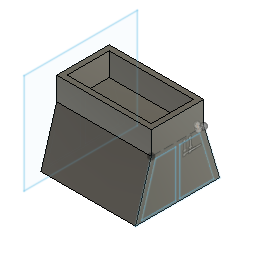
creality-ender-3-v2-foot-extender (Autodesk Fusion 360 design; units mm, degrees)
Autodesk Fusion 360 part; units mm, degrees
sketch "Sketch1" plane through (0, 0, 0) normal (0, 0, 1) x (1, 0, 0)
  line L0 (20, -10) -> (-20, -10)
  line L1 (-20, -10) -> (-20, 10)
  line L2 (-20, 10) -> (20, 10)
  line L3 (20, 10) -> (20, -10)
  line L4 (20, -10) -> (-20, 10) construction
  line L5 (-20, -10) -> (20, 10) construction
  line L6 (22.5, -12.5) -> (-22.5, -12.5)
  line L7 (-22.5, -12.5) -> (-22.5, 12.5)
  line L8 (-22.5, 12.5) -> (22.5, 12.5)
  line L9 (22.5, 12.5) -> (22.5, -12.5)
  line L10 (22.5, -12.5) -> (-22.5, 12.5) construction
  line L11 (-22.5, -12.5) -> (22.5, 12.5) construction
  dimension "d1" = 40
  dimension "d2" = 20
  dimension "d3" = 45
  dimension "d4" = 25
  constraint horizontal L0
  constraint perpendicular L0 L1
  constraint parallel L0 L2
  constraint parallel L1 L3
  constraint coincident L4 origin
  constraint coincident L5 origin
  constraint horizontal L6
  constraint perpendicular L6 L7
  constraint parallel L6 L8
  constraint parallel L7 L9
  constraint coincident L10 origin
  constraint coincident L11 origin
  measures "d1" distance of L1.end L2.end
  measures "d2" distance of L0.end L1.end
  measures "d3" distance of L7.end L8.end
  measures "d4" distance of L6.end L7.end
extrude "Extrude1" add sketch "Sketch1" along normal blind 11 makes body 1
sketch "Sketch4" plane through (22.5, 0, 0) normal (1, 0, 0) x (0, 1, 0)
  line L0 (-12.5, 0) -> (12.5, 0)
  line L1 (12.5, 0) -> (12.5, 11)
  line L2 (12.5, 11) -> (-12.5, 11)
  line L3 (-12.5, 11) -> (-12.5, 0)
  line L4 (-12.5, 0) -> (12.281, 0) construction
  line L5 (-12.5, 0) -> (-20, -25)
  line L6 (-20, -25) -> (20, -25)
  line L7 (20, -25) -> (12.5, 0)
  line L8 (12.5, 0) -> (20, -25) construction
  line L9 (12.281, -0.0657) -> (12.5, 0) construction
  line L10 (-12.5, 0) -> (-20, -25) construction
  line L11 (17.0904, -24.0014) -> (10.4521, -1.8738)
  line L12 (-17.0895, -23.9987) -> (-10.4636, -1.8738) construction
  line L13 (-1, -1.8738) -> (-1, -24)
  line L14 (1, -24.0002) -> (1, -1.8738)
  line L15 (-17.0895, -23.9987) -> (-1, -24)
  line L16 (1, -24.0002) -> (17.0904, -24.0014)
  line L17 (17.0904, -24.0014) -> (10.4521, -1.8738) construction
  line L18 (9.8899, 0) -> (9.2425, 2.1581) construction
  line L19 (-17.0895, -23.9987) -> (-10.4636, -1.8738)
  line L20 (-10.4636, -1.8738) -> (-1, -1.8738)
  line L21 (1, -1.8738) -> (10.4521, -1.8738)
  constraint horizontal L4
  constraint coincident L0.start L3.end
  constraint coincident L0.end L1.start
  constraint perpendicular L4 L14
  constraint collinear L15 L16
  constraint coincident L4 L18.start
  constraint collinear L17 L18
  constraint horizontal L20
  constraint coincident L14.end L20
  constraint collinear L20 L21
  constraint vertical L13
extrude "Extrude10" add sketch "Sketch4" against normal blind 2 separate body contours L11 L14 L16 L21 | L13 L15 L19 L20 makes body 2 at (22.5, 9.5141, -16.6251) makes body 3 at (22.5, -9.5177, -16.6242)
extrude "Extrude8" add sketch "Sketch4" against normal up to surface (45 mm away) contours L0 L5 L6 L7 bodies 1
sketch "Sketch9" plane through (0, 0, -1.8738) normal (0, 0, -1) x (1, 0, 0)
  line L0 (-22.5, 10.4636) -> (-22.5, 1)
  line L1 (-22.5, 1) -> (22.5, 1)
  line L2 (22.5, 1) -> (22.5, 10.4636)
  line L3 (22.5, 10.4636) -> (-22.5, 10.4636)
  line L4 (-1, 20) -> (1, 20)
  line L5 (1, 20) -> (1, -20)
  line L6 (1, -20) -> (-1, -20)
  line L7 (-1, -20) -> (-1, 20)
  line L8 (-22.5, 19) -> (-21.5, 20)
  line L9 (-21.5, 20) -> (-2, 0.5)
  line L10 (-2, 0.5) -> (-3, -0.5)
  line L11 (-3, -0.5) -> (-22.5, 19)
  line L12 (-22.5, -19) -> (-21.5, -20)
  line L13 (-21.5, -20) -> (-2, -0.5)
  line L14 (-2, -0.5) -> (-3, 0.5)
  line L15 (-3, 0.5) -> (-22.5, -19)
  line L16 (22.5, -19) -> (21.5, -20)
  line L17 (21.5, -20) -> (1.9964, -0.4964)
  line L18 (1.9964, -0.4964) -> (2.9964, 0.5036)
  line L19 (2.9964, 0.5036) -> (22.5, -19)
  line L20 (21.5, 20) -> (22.5, 19)
  line L21 (22.5, 19) -> (2.5, -1)
  line L22 (2.5, -1) -> (1.5, 0)
  line L23 (1.5, 0) -> (21.5, 20)
  constraint horizontal L4
  constraint vertical L5
  constraint horizontal L6
  constraint vertical L7
  constraint perpendicular L8 L9
  constraint parallel L8 L10
  constraint parallel L9 L11
  constraint perpendicular L12 L13
  constraint parallel L12 L14
  constraint parallel L13 L15
  constraint perpendicular L10 L12
  constraint perpendicular L16 L17
  constraint parallel L16 L18
  constraint parallel L17 L19
  constraint parallel L10 L16
  constraint perpendicular L20 L21
  constraint parallel L20 L22
  constraint parallel L21 L23
  constraint parallel L19 L20
extrude "Extrude9" add sketch "Sketch9" along normal up to surface (23.1262 mm away) contours L3 L8 L9 L11 | L1 L3 L9 L11 | L1 L9 L10 L11 L14 L15 | L10 L11 L14 L15 | L10 L11 L12 L13 L14 L15 | L3 L4 L5 L7 | L1 L3 L5 L7 | L1 L5 L6 L7 | L3 L20 L21 L23 | L1 L3 L21 L23 | L1 L18 L19 L21 L22 L23 | L17 L18 L19 L21 L22 | L16 L17 L19 L21 bodies 1
sketch "Sketch10" plane through (-22.5, 0, 0) normal (-1, 0, 0) x (0, -1, 0)
  line L0 (-1, -1.8738) -> (-1, -24.0002)
  line L1 (-1, -24.0002) -> (-17.0904, -24.0014)
  line L2 (-17.0904, -24.0014) -> (-10.4521, -1.8738)
  line L3 (-10.4521, -1.8738) -> (-1, -1.8738)
  line L4 (10.4636, -1.8738) -> (17.0895, -23.9987)
  line L5 (17.0895, -23.9987) -> (1, -24)
  line L6 (1, -24) -> (1, -1.8738)
  line L7 (1, -1.8738) -> (10.4636, -1.8738)
  line L8 (-19, -21.6667) -> (-20, -25)
  line L9 (-20, -25) -> (20, -25)
  line L10 (20, -25) -> (19, -21.6667)
  line L11 (19, -21.6667) -> (12.5, 0)
  line L12 (12.5, 0) -> (12.5, 11)
  line L13 (12.5, 11) -> (-12.5, 11)
  line L14 (-12.5, 11) -> (-12.5, 0)
  line L15 (-12.5, 0) -> (-19, -21.6667)
  line L16 (-25.8354, 18.4889) -> (28, 18.4889)
  line L17 (28, 18.4889) -> (28, -29)
  line L18 (28, -29) -> (-25.8354, -29)
  line L19 (-25.8354, -29) -> (-25.8354, 18.4889)
  constraint horizontal L16
  constraint vertical L17
  constraint horizontal L18
  constraint vertical L19
extrude "Extrude12" cut sketch "Sketch10" against normal blind 74 contours L16 L17 L18 L19 bodies 1
extrude "Extrude11" add sketch "Sketch10" against normal blind 2 contours L0 L1 L2 L3 | L4 L5 L6 L7 bodies 1
combine "Combine2" operation add target body 1 tool bodies 2 3
equation "d3 = 40 mm + 5 mm"
equation "d4 = 20 mm + 5 mm"
